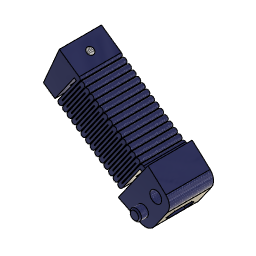
Tibia feet spring support v7 (Autodesk Fusion 360 design; units mm, degrees)
Autodesk Fusion 360 part; units mm, degrees
sketch "Sketch1" plane through (0, 0, 0) normal (0, 1, 0) x (1, 0, 0)
  arc A0 (37.3, 10) -> (161.7212, 42.0206) centre (37.3, 267.7398) ccw
  circle A1 centre (0, 0) radius 2.5
  arc A2 (37.3, -10) -> (167.1141, 34.3187) centre (37.3, 202.279) ccw
  line L0 (76.2246, 12.9562) -> (80.0659, -5.6475)
  line L1 (-10.1, -10) -> (29.9, -10)
  line L2 (-17.5, 10) -> (-10.1, 10)
  line L3 (-17.5, -10) -> (-17.5, 10)
  line L4 (-10.1, 10) -> (-10.1, -10)
  line L5 (-10.1, -10) -> (-17.5, -10)
  line L6 (37.3, -10) -> (37.3, 10)
  line L7 (161.7212, 42.0206) -> (167.1141, 34.3187)
  line L8 (38.4, -18.5) -> (38.4, 18.5) construction
  line L9 (-10.1, 10) -> (-10.1, -10)
  line L10 (-18.6, 18.5) -> (-18.6, -18.5)
  line L11 (169.6952, 30.6325) -> (169.9824, 51.1436) construction
  line L12 (29.9, -10) -> (37.3, -10)
  line L13 (159.1401, 45.7067) -> (178.5861, 38.8564) construction
  line L14 (29.9, 10) -> (29.9, -10)
  line L15 (80.0659, -5.6475) -> (84.1183, 14.2879) construction
  line L16 (84.1183, 14.2879) -> (87.8714, -3.8882)
  line L17 (-18.6, -18.5) -> (38.4, -18.5)
  arc A3 (38.4, 18.5) -> (169.9824, 51.1436) centre (38.4, 300.018) ccw
  line L18 (-17.5, -10) -> (-18.6, -10)
  line L19 (37.3, 10) -> (29.9, 10)
  line L20 (38.4, 18.5) -> (-18.6, 18.5)
  arc A4 (38.4, -18.5) -> (178.5861, 38.8564) centre (38.4, 181.4943) ccw
  line L21 (-17.5, 10) -> (-18.6, 10)
  line L22 (29.9, 10) -> (-10.1, 10)
  line L23 (9.9, -10) -> (9.9, -18.5) construction
  line L24 (0, 0) -> (174.2843, 45) construction
  line L25 (118.3255, 23.0672) -> (124.5058, 8.7395)
  line L26 (124.5058, 8.7395) -> (125.8994, 25.7068) construction
  line L27 (9.9, 10) -> (9.9, 18.5) construction
  line L28 (125.8994, 25.7068) -> (131.7408, 12.165)
  line L29 (159.1401, 45.7067) -> (169.6952, 30.6325) construction
  line L30 (29.9, -10) -> (29.9, 10)
  line L31 (169.9824, 51.1436) -> (178.5861, 38.8564)
  line L32 (174.2843, 45) -> (122.8386, 8.9774) construction
  line L33 (168.4695, 32.383) -> (167.0359, 31.3793)
  line L34 (167.0359, 31.3793) -> (160.153, 41.2091)
  line L35 (160.153, 41.2091) -> (159.9482, 41.0657)
  line L36 (167.3223, 34.0213) -> (166.5032, 33.4477)
  line L37 (166.5032, 33.4477) -> (159.6202, 43.2776)
  line L38 (159.6202, 43.2776) -> (158.1867, 42.2738)
  line L39 (159.9482, 41.0657) -> (166.8312, 31.2359)
  line L40 (158.1867, 42.2738) -> (165.0696, 32.444)
  line L41 (165.0696, 32.444) -> (164.9672, 32.3723)
  line L42 (164.9672, 32.3723) -> (166.1144, 30.734)
  line L43 (166.1144, 30.734) -> (166.8312, 31.2359)
  line L44 (161.7212, 42.0206) -> (159.1401, 45.7067)
  line L45 (167.1141, 34.3187) -> (169.6952, 30.6325)
  line L46 (166.6056, 33.5194) -> (167.7527, 31.8811)
  circle A5 centre (165.6125, 31.4507) radius 0.875
  circle A6 centre (167.2508, 32.5979) radius 0.875
  circle A7 centre (159.4054, 42.0589) radius 0.875
  circle A8 centre (160.1223, 41.035) radius 0.125
  circle A9 centre (166.5339, 33.6218) radius 0.125
  circle A10 centre (164.8955, 32.4747) radius 0.125
  line L47 (133.5628, 7.9411) -> (127.9007, 21.0673)
  line L48 (127.9007, 21.0673) -> (136.172, 26.8589)
  line L49 (136.172, 26.8589) -> (144.2021, 15.3908)
  line L50 (144.2021, 15.3908) -> (133.5628, 7.9411)
  line L51 (144.2021, 15.3908) -> (144.8164, 15.821)
  line L52 (144.8164, 15.821) -> (143.6693, 17.4593)
  line L53 (143.6693, 17.4593) -> (143.0549, 17.0291)
  line L54 (137.7449, 10.8695) -> (132.0829, 23.9957)
  point P0 (169.8534, 41.9327)
  point P1 (9.9, 13.85)
  point P2 (9.9, -13.85)
  point P3 (174.2843, 45)
  point P4 (82.0921, 4.3202)
  point P5 (125.2026, 17.2232)
  point P6 (37.3, 0)
  point P7 (159.1401, 45.7067)
  dimension "d1" = 5
  dimension "d2" = 10.1
  dimension "d3" = 40
  dimension "d4" = 20
  dimension "d5" = 10
  dimension "d6" = 7.4
  dimension "d7" = 8.5
  dimension "d8" = 8.5
  dimension "d9" = 8.5
  dimension "d10" = 8.5
  dimension "d11" = 180
  dimension "d12" = 45
  dimension "d13" = 35
  dimension "d14" = 15
  dimension "d15" = 12
  dimension "d16" = 4.5
  dimension "d17" = 4.5
  dimension "d18" = 8
  dimension "d19" = 8
  dimension "d20" = 45
  dimension "d21" = 45
  dimension "d22" = 11.667
  dimension "d23" = 11.667
  dimension "d24" = 27.7
  dimension "d25" = 13.85
  dimension "d26" = 2
  dimension "d29" = 7
  dimension "d30" = 7
  dimension "d31" = 2
  dimension "d32" = 0.25
  dimension "d33" = 1.75
  dimension "d34" = 0.875
  dimension "d35" = 0.875
  dimension "d37" = 1
  dimension "d38" = 0.125
  dimension "d39" = 1.75
  dimension "d53" = 0.75
  dimension "d54" = 26
  dimension "d66" = 5
  constraint coincident A1.centre L24.start
  constraint horizontal L1
  constraint vertical L30
  constraint horizontal L22
  constraint vertical L4
  constraint horizontal L5
  constraint vertical L3
  constraint horizontal L2
  constraint vertical L9
  constraint horizontal L12
  constraint vertical L6
  constraint horizontal L19
  constraint vertical L14
  constraint coincident L2.end L4.start
  constraint coincident L14.start L19.end
  constraint equal L5 L12
  constraint horizontal L17
  constraint vertical L8
  constraint horizontal L20
  constraint vertical L10
  constraint coincident P3 L31
  constraint tangent L17 A4
  constraint tangent A3 L20
  constraint midpoint P3 L31
  constraint coincident P3 L24.end
  constraint parallel L29 L31
  constraint coincident A2.end L29
  constraint tangent A2 L12
  constraint coincident A0.end L29
  constraint tangent A0 L19
  constraint coincident L11.start A4
  constraint coincident P7 A3
  constraint coincident L0.start A0
  constraint coincident L0.end A2
  constraint coincident L15.end A0
  constraint coincident L16.end A2
  constraint parallel L0 L16
  constraint coincident L25.start A0
  constraint coincident L25.end A2
  constraint coincident L26.end A0
  constraint coincident L28.end A2
  constraint parallel L25 L28
  constraint midpoint P4 L15
  constraint midpoint P5 L26
  constraint midpoint P6 L6
  constraint coincident L18.end L10
  constraint perpendicular L10 L18
  constraint coincident L21.end L10
  constraint perpendicular L10 L21
  constraint midpoint L23.start L1
  constraint midpoint L23.end L17
  constraint midpoint L27.start L22
  constraint midpoint L27.end L20
  constraint coincident P0 L13
  constraint coincident P0 L11
  constraint coincident P1 L27
  constraint perpendicular L29 L32
  constraint coincident L29 L33.start
  constraint perpendicular L29 L33
  constraint perpendicular L32 L34
  constraint perpendicular L34 L35
  constraint coincident L29 L36.start
  constraint perpendicular L29 L36
  constraint perpendicular L37 L38
  constraint perpendicular L32 L37
  constraint perpendicular L35 L39
  constraint perpendicular L38 L40
  constraint perpendicular L40 L41
  constraint perpendicular L39 L43
  constraint collinear L33 L43
  constraint collinear L36 L41
  constraint perpendicular L42 L43
  constraint coincident L36 L46.start
  constraint coincident L33 L46.end
  constraint perpendicular L33 L46
  constraint tangent L39 A5
  constraint tangent L43 A5
  constraint tangent L34 A6
  constraint tangent L33 A6
  constraint equal A5 A6
  constraint tangent L37 A7
  constraint tangent L38 A7
  constraint tangent L40 A7
  constraint tangent L34 A8
  constraint tangent L39 A8
  constraint tangent L35 A8
  constraint tangent L36 A9
  constraint tangent L37 A9
  constraint equal A8 A9
  constraint tangent L40 A10
  constraint tangent L41 A10
  constraint equal A9 A10
  constraint parallel L32 L50
  constraint parallel L32 L48
  constraint parallel L40 L49
  constraint coincident L28.end L47
  constraint coincident L26.end L47
  constraint coincident L49 L50.start
  constraint perpendicular L49 L51
  constraint perpendicular L51 L52
  constraint coincident L49 L53.end
  constraint perpendicular L49 L53
  constraint collinear L43 L51
  constraint collinear L41 L53
  constraint collinear L43 L50
  constraint coincident P7 L13.start
  constraint collinear L38 L48
  constraint coincident L50 L54.start
  constraint parallel L28 L54
  constraint coincident L48 L54.end
  measures "d1" diameter of A1
  measures "d2" distance of A1.centre L4
  measures "d3" distance of L1.start L1.end
  measures "d4" distance of L14.start L1.end
  measures "d5" distance of A1.centre L1
  measures "d6" distance of L1.start L3.start
  measures "d7" distance of L9 L10
  measures "d8" distance of L8 L30
  measures "d9" distance of L20 L22
  measures "d10" distance of L1 L17
  measures "d11" distance of A1.centre P3
  measures "d12" vertical distance of P3 A1.centre
  measures "d13" angle of L10 L31
  measures "d14" distance of L13.end L11.end
  measures "d15" distance of L29 L31
  measures "d16" distance of L11.start A2.end
  measures "d17" distance of P7 A0.end
  measures "d18" distance of L0 L16
  measures "d19" distance of L25 L28
  measures "d20" distance of P4 P6
  measures "d21" distance of P4 P5
  measures "d22" angle of L0 L6
  measures "d23" angle of L16 L25
  measures "d24" distance of P1 P2
  measures "d25" vertical distance of A1.centre P1
  measures "d26" distance of L33 L36
  measures "d29" distance of L32 L33
  measures "d30" distance of L32 L38
  measures "d31" distance of L35 L38
  measures "d32" distance of L34 L39
  measures "d33" distance of L37.end L38.end
  measures "d34" distance of L39.end L42.end
  measures "d35" distance of L34 L46
  measures "d37" distance of L7 L37
  measures "d38" distance of L37 L46
  measures "d39" diameter of A6
  measures "d53" distance of L49.end L51.end
  measures "d54" distance of L42 L52
  measures "d66" distance of L47 L54
extrude "Extrude1" add sketch "Sketch1" along normal mid plane 15.75 contours L7 A3 A4 L31 L44 L45
fillet "Fillet1" radius 4 2 edges at (178.5861, 0, -38.8564) (169.9824, 0, -51.1436)
extrude "Extrude2" add sketch "Sketch1" along normal mid plane 15 contours L33 L45 A6 | L46 A6 | L36 L45 L46 A6 picked at (167.6154, 32.7553)
extrude "Extrude3" add sketch "Sketch1" along normal mid plane 15 contours A0 L34 L35 L37 L39 L40 A7 | A0 A2 L39 L40 | A0 L35 L39 A8 | A0 L39 A8 | A7 | A2 L39 L40 L41 L42 A5 | L40 L41 A10 | A0 L34 L35 A8 | A0 L34 A8 | A0 A2 L34 L37 | A2 L34 L36 L37 L46 A6 | L42 A5 | L46 A6 | L36 L37 A9 picked at (165.9983, 31.7152) picked at (166.8361, 32.3549)
pattern_linear "R-Pattern1" count 14 spacing 2 along (-0.819152, 0, 0.573576) of "Extrude3"
extrude "Extrude4" add sketch "Sketch1" along normal mid plane 15 contours A2 L48 L49 L54 | A2 L49 L50 L54 | L49 L51 L52 L53
sketch "Sketch2" plane through (138.0896, 0, -96.6914) normal (0.819152, 0, -0.573576) x (0, 1, 0)
  line L0 (-7.875, 59.112) -> (7.875, 59.112)
  line L1 (7.875, 59.112) -> (7.875, 67.1879)
  line L2 (7.875, 67.1879) -> (-7.875, 67.1879)
  line L3 (-7.875, 67.1879) -> (-7.875, 59.112)
  line L4 (-3, 63.362) -> (3, 63.362)
  line L5 (3, 63.362) -> (3, 59.362)
  line L6 (3, 59.362) -> (-3, 59.362)
  line L7 (-3, 59.362) -> (-3, 63.362)
  line L8 (3, 63.362) -> (5, 61.362)
  line L9 (5, 61.362) -> (3, 59.362)
  line L10 (-3, 63.362) -> (-5, 61.362)
  line L11 (-5, 61.362) -> (-3, 59.362)
  line L12 (-6.0161, 61.362) -> (6.3975, 61.362) construction
  line L13 (0, 64.8024) -> (0, 57.8612) construction
  dimension "d57" = 2
  dimension "d58" = 10
  dimension "d59" = 4
  dimension "d60" = 7.875
  dimension "d61" = 5
  dimension "d82" = 0.25
  constraint horizontal L4
  constraint vertical L5
  constraint horizontal L6
  constraint vertical L7
  constraint parallel L9 L10
  constraint parallel L8 L11
  constraint perpendicular L5 L12
  constraint coincident L8.end L12
  constraint coincident L10.end L12
  constraint perpendicular L6 L13
  measures "d57" distance of L5 L8.end
  measures "d58" distance of L8.end L10.end
  measures "d59" distance of L4.end L5.end
  measures "d60" distance of L3 L13
  measures "d61" distance of L10.end L13
  measures "d82" distance of L0 L6
extrude "Extrude5" cut sketch "Sketch2" against normal blind 63 contours L4 L5 L6 L7 | L7 L10 L11 | L5 L8 L9
sketch "Sketch3" plane through (0, -7.875, 0) normal (0, -1, 0) x (1, 0, 0)
  arc A0 (166.8925, -49.5344) -> (171.9948, -48.2696) centre (168.7182, -45.9753) ccw
  line L0 (171.9948, -48.2696) -> (176.627, -41.6543)
  arc A1 (176.627, -41.6543) -> (176.1045, -36.4592) centre (173.3503, -39.36) ccw
  arc A2 (176.1045, -36.4592) -> (169.6952, -30.6325) centre (38.4, -181.4943) ccw
  line L1 (169.6952, -30.6325) -> (159.1401, -45.7067)
  arc A3 (166.8925, -49.5344) -> (159.1401, -45.7067) centre (38.4, -300.018) ccw
  circle A4 centre (172.4831, -38.8551) radius 2.1
  circle A5 centre (167.8943, -45.4086) radius 2
  line L2 (167.8943, -45.4086) -> (172.4831, -38.8551) construction
  line L3 (164.4176, -38.1696) -> (174.3109, -44.9619) construction
  dimension "d67" = 4
  dimension "d68" = 5
  dimension "d69" = 4
  dimension "d70" = 4
  dimension "d71" = 4.2
  constraint coincident A5.centre L2.start
  constraint coincident A4.centre L2.end
  constraint parallel L1 L2
  constraint midpoint L1 L3.start
  constraint midpoint L0 L3.end
  measures "d67" diameter of A5
  measures "d68" distance of L0 A5.centre
  measures "d69" distance of A5.centre L3
  measures "d70" distance of A4.centre L3
  measures "d71" diameter of A4
extrude "Extrude6" cut sketch "Sketch3" against normal through all contours A4
extrude "Extrude7" add sketch "Sketch3" along normal blind 3 contours A5
chamfer "Chamfer1" distance 0.5 angle 45 1 edges at (166.0296, -10.875, -46.1318)
mirror "Mirror1" about plane through (0, 0, 0) normal (0, 1, 0) of "Extrude7", "Chamfer1"
sketch "Sketch5" plane through (40.2097, 0, 57.4254) normal (0.573576, 0, 0.819152) x (0, 1, 0)
  line L0 (-7.5, -127.7012) -> (7.5, -127.7012)
  line L1 (7.5, -127.7012) -> (7.5, -119.0685)
  line L2 (7.5, -119.0685) -> (-7.5, -119.0685)
  line L3 (-7.5, -119.0685) -> (-7.5, -127.7012)
  line L4 (7.5, -119.0685) -> (-7.5, -127.7012) construction
  line L5 (7.5, -127.7012) -> (-7.5, -119.0685) construction
  point P0 (0, -123.3849)
  constraint coincident L1.end L2.start
  constraint coincident L0.start L3.end
  constraint coincident L0.end L1.start
  constraint coincident L2.end L3.start
  constraint midpoint L5 P0
hole "Hole1" at (141.2807, 0, -13.3452) direction (-0.573576, 0, -0.819152) diameter 2.529 end up to surface (6.7415 mm away)
thread "Thread1" "ISO Metric profile 3.0 M3x0.5 6H" major diameter 3.086 minor diameter 2.529 pitch 0.5 angle 60 resizes the face on face at (139.3663, 1.008, -14.7481)
equation "d31 = d26"
equation "d34 = d33 / 2"
equation "d35 = d34"
equation "d38 = d32 / 2"
equation "d39 = d35 * 2"
equation "d60 = ( 15.75 / 2 ) * 1 mm"
